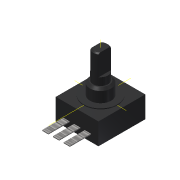
# Autodesk Inventor part: empty
Saved by Autodesk Inventor 2014 (Build 180170000, 170)
## iProperties
Created: 2015-04-13
Part Number: empty
Material: Generic
Document SubType Name: Modeling
Designer: Martin
Density: 1 g/cm^3
Appearance: Default
Author: Martin
Autodesk Inventor part; units mm, degrees
ref_plane "YZ Plane" through (0, 0, 0) normal (1, 0, 0) x (0, 1, 0)
ref_plane "XZ Plane" through (0, 0, 0) normal (0, 1, 0) x (-1, 0, 0)
ref_plane "XY Plane" through (0, 0, 0) normal (0, 0, 1) x (1, 0, 0)
sketch "Sketch1" plane through (0, 0, 0) normal (0, 0, 1) x (1, 0, 0)
  line L0 (-5.05, -5.55) -> (5.05, -5.55)
  line L1 (5.05, -5.55) -> (5.05, 5.55)
  line L2 (5.05, 5.55) -> (-5.05, 5.55)
  line L3 (-5.05, 5.55) -> (-5.05, -5.55)
  line L4 (-5.05, -5.55) -> (5.05, 5.55) construction
  line L5 (5.05, -5.55) -> (-5.05, 5.55) construction
  point P0 (0, 0)
  dimension "d0" = 10.1
  dimension "d1" = 11.1
  constraints: 12 end point, 2 midpoint, 2 parallel, 1 horizontal, 1 perpendicular
  measures "d0" distance of L1.end L2.end
  measures "d1" distance of L0.end L1.end
extrude "Extrusion1" add sketch "Sketch1" against normal blind 5.1
sketch "Sketch2" plane through (0, 0, 0) normal (1, 0, 0) x (0, 1, 0)
  line L0 (-7.77, 0) -> (7.77, 0) projected
  line L1 (0, -6.12) -> (0, 1.02) projected
  line L2 (0, 0) -> (0, 22.7179)
  line L3 (0, 0) -> (4, 0)
  line L4 (4, 0) -> (4, 0.2)
  line L5 (4, 0.2) -> (2.5, 0.2)
  line L6 (2.5, 0.2) -> (2.5, 3.2)
  line L7 (2.5, 3.2) -> (1.75, 3.2)
  line L8 (1.75, 3.2) -> (1.75, 9.9)
  line L9 (1.75, 9.9) -> (0, 9.9)
  line L10 (0, 9.9) -> (0, 0)
  line L11 (5.55, -5.1) -> (-5.55, -5.1) projected
  dimension "d4" = 8
  dimension "d5" = 5
  dimension "d6" = 3.5
  dimension "d7" = 5.3
  dimension "d8" = 8.3
  dimension "d9" = 15
  constraints: 18 end point, 3 parallel, 3 perpendicular, 3 point on line, 1 collinear
  measures "d4" diameter of L4 L2
  measures "d5" diameter of L6 L2
  measures "d6" diameter of L8 L2
  measures "d7" distance between parallel lines of L11 L5
  measures "d8" distance between parallel lines of L11 L7
  measures "d9" distance between parallel lines of L11 L9
revolve "Revolution1" add sketch "Sketch2" angle 360 about axis through (0, 0, 0) along (0, 0, 1)
chamfer "Chamfer1" distance 0.5 angle 45 1 edges at (0, -2.5, 3.2)
sketch "Sketch3" plane through (0, 0, 9.9) normal (0, 0, 1) x (1, 0, 0)
  circle A0 centre (0, 0) radius 1.75 projected
  line L0 (0, -7.77) -> (0, 7.77) projected
  line L1 (-1, 1.4361) -> (-1, -1.4361)
  line L2 (1, 1.4361) -> (1, -1.4361)
  dimension "d14" = 2
  constraints: 4 end point, 4 point on circle, 1 parallel, 1 other
  measures "d14" distance between parallel lines of L2 L1
extrude "Extrusion2" cut sketch "Sketch3" against normal blind 4.9 contours A0 L2 | L1 A0
chamfer "Chamfer2" distance 0.25 angle 45 3 edges at (0, -1.75, 9.9) (-0.524, 1.6697, 9.9) (0.524, 1.6697, 9.9)
sketch "Sketch4" plane through (0, 0, 0) normal (1, 0, 0) x (0, 1, 0)
  line L0 (-5.55, 0) -> (-5.55, -5.1) projected
  line L1 (-5.55, -3.6) -> (-10.55, -3.6)
  line L2 (-10.55, -3.4) -> (-5.55, -3.4)
  line L3 (-5.55, -3.4) -> (-5.55, -3.6)
  line L4 (5.55, -5.1) -> (-5.55, -5.1) projected
  line L5 (-10.55, -3.4) -> (-10.55, -3.6)
  point P0 (0, 0)
  dimension "d22" = 1.5
  dimension "d29" = 0.2
  dimension "d30" = 5
  constraints: 8 end point, 3 perpendicular, 2 point on line, 1 collinear
  measures "d22" distance between parallel lines of L4 L1
  measures "d29" distance between parallel lines of L1 L2
  measures "d30" distance of L2.start L2.end
extrude "Extrusion3" add sketch "Sketch4" along normal mid plane 1.48
pattern_linear "Rectangular Pattern1" count 3 spacing 2.54 along (1, 0, 0) of "Extrusion3" first direction both ways yes
body "Solid1"
